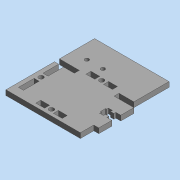
# Autodesk Inventor part: X-Anchor_Side
Saved by Autodesk Inventor 2016 SP1 (Build 200210100, 210)
## iProperties
Created: 2015-12-01
Part Number: X-Anchor_Side
Material: Generic
Document SubType Name: Modeling
Designer: Mohamed A.
Density: 1 g/cm^3
Appearance: Default
Author: Mohamed A.
Autodesk Inventor part; units mm, degrees
ref_plane "YZ Plane" through (0, 0, 0) normal (1, 0, 0) x (0, 1, 0)
ref_plane "XZ Plane" through (0, 0, 0) normal (0, 1, 0) x (-1, 0, 0)
ref_plane "XY Plane" through (0, 0, 0) normal (0, 0, 1) x (1, 0, 0)
sketch "Sketch1" plane through (0, 0, 0) normal (0, 0, 1) x (1, 0, 0)
  line L0 (0, 0) -> (47.5, 0)
  line L1 (47.5, 0) -> (47.5, 37)
  line L2 (47.5, 37) -> (0, 37)
  line L3 (0, 37) -> (0, 0)
  dimension "d60" = 47.5
  dimension "d61" = 37
  constraints: 8 end point, 2 parallel, 1 horizontal, 1 perpendicular
  measures "d60" distance between parallel lines of L1 L3
  measures "d61" distance between parallel lines of L0 L2
extrude "Extrusion1" add sketch "Sketch1" against normal blind 3
sketch "Sketch6" plane through (0, 0, 0) normal (0, 0, 1) x (1, 0, 0)
  line L0 (47.5, 0) -> (47.5, 37) projected
  line L1 (47.5, 37) -> (0, 37) projected
  line L2 (0, 37) -> (47.5, 37) projected
  line L3 (47.5, 37) -> (44.5, 37)
  line L4 (44.5, 37) -> (44.5, 29)
  line L5 (44.5, 29) -> (47.5, 29)
  line L6 (47.5, 29) -> (47.5, 37)
  line L7 (44.5, 0) -> (44.5, 8)
  line L8 (44.5, 8) -> (47.5, 8)
  line L9 (47.5, 8) -> (47.5, 0)
  line L10 (47.5, 0) -> (44.5, 0)
  line L11 (-10.772, 18.5) -> (61.9279, 18.5) construction
  line L12 (23.75, 42.476) -> (23.75, -8.8223) construction
  line L13 (47.5, 20) -> (39.5, 20)
  line L14 (39.5, 20) -> (39.5, 17)
  line L15 (39.5, 17) -> (47.5, 17)
  line L16 (47.5, 17) -> (47.5, 20)
  line L17 (47.5, 37) -> (47.5, 0) projected
  line L18 (44.5, 21.15) -> (47.5, 21.15)
  line L19 (47.5, 21.15) -> (47.5, 15.85)
  line L20 (47.5, 15.85) -> (44.5, 15.85)
  line L21 (44.5, 15.85) -> (44.5, 21.15)
  line L22 (40.1, 21.15) -> (42.5, 21.15)
  line L23 (42.5, 21.15) -> (42.5, 15.85)
  line L24 (42.5, 15.85) -> (40.1, 15.85)
  line L25 (40.1, 15.85) -> (40.1, 21.15)
  line L26 (15.8333, 35) -> (21.1, 35)
  line L27 (31.6667, 35) -> (31.6667, 32)
  line L28 (31.6667, 32) -> (26.4, 32)
  line L29 (15.8333, 32) -> (15.8333, 35)
  line L30 (26.4, 35) -> (26.4, 32)
  line L31 (21.1, 32) -> (21.1, 35)
  line L32 (26.4, 35) -> (31.6667, 35)
  line L33 (21.1, 32) -> (15.8333, 32)
  circle A0 centre (23.75, 33.5) radius 1.4
  line L34 (0, 0) -> (47.5, 0) projected
  line L35 (0, 0) -> (0, 37) projected
  line L36 (0, 32) -> (11.875, 32)
  line L37 (11.875, 32) -> (11.875, 29)
  line L38 (11.875, 29) -> (0, 29)
  line L39 (0, 29) -> (0, 32)
  line L40 (44.5, 32) -> (35.625, 32)
  line L41 (35.625, 32) -> (35.625, 29)
  line L42 (35.625, 29) -> (44.5, 29)
  line L43 (44.5, 29) -> (44.5, 32)
  line L44 (15.8333, 2) -> (21.1, 2)
  line L45 (31.6667, 2) -> (31.6667, 5)
  line L46 (31.6667, 5) -> (26.4, 5)
  line L47 (15.8333, 5) -> (15.8333, 2)
  line L48 (26.4, 2) -> (26.4, 5)
  line L49 (21.1, 5) -> (21.1, 2)
  line L50 (26.4, 2) -> (31.6667, 2)
  line L51 (21.1, 5) -> (15.8333, 5)
  circle A1 centre (23.75, 3.5) radius 1.4
  line L52 (5.5, 19.65) -> (2.5, 19.65)
  line L53 (2.5, 19.65) -> (2.5, 29)
  line L54 (2.5, 29) -> (5.5, 29)
  line L55 (5.5, 29) -> (5.5, 19.65)
  line L56 (2.5, 14.35) -> (5.5, 14.35)
  line L57 (5.5, 14.35) -> (5.5, 5)
  line L58 (5.5, 5) -> (2.5, 5)
  line L59 (2.5, 5) -> (2.5, 14.35)
  circle A2 centre (4, 17) radius 1.4
  dimension "d65" = 3
  dimension "d75" = 8
  dimension "d76" = 3
  dimension "d78" = 5.3
  dimension "d80" = 5
  dimension "d81" = 2.4
  dimension "d83" = 3
  dimension "d84" = 15.8333
  dimension "d85" = 2
  dimension "d86" = 5.3
  dimension "d87" = 2.8
  dimension "d88" = 3
  dimension "d89" = 23.75
  dimension "d90" = 47.5
  dimension "d91" = 2.8
  dimension "d92" = 5.3
  dimension "d93" = 2.65
  dimension "d94" = 1.5
  constraints: 108 end point, 20 parallel, 15 horizontal, 9 symmetric about line, 8 collinear, 8 point on line, 7 perpendicular, 6 vertical, 3 centre point, 16 other
  measures "d65" distance of L5.end L4.end
  measures "d75" distance of L15.end L14.end
  measures "d76" distance of L14.end L13.end
  measures "d78" distance between parallel lines of L20 L18
  measures "d80" distance between parallel lines of L0 L23
  measures "d81" distance between parallel lines of L25 L23
  measures "d83" distance of L27.start L27.end
  measures "d84" distance between parallel lines of L27 L29
  measures "d85" distance between parallel lines of L26 L1
  measures "d86" distance of L28.end L31.start
  measures "d87" diameter of A0
  measures "d88" distance of L36.end L37.end
  measures "d89" distance between parallel lines of L41 L37
  measures "d90" distance between parallel lines of L0 L35
  measures "d91" diameter of A2
  measures "d92" distance between parallel lines of L52 L56
  measures "d93" distance from line of A2.centre L56
  measures "d94" distance from line of L59 A2.centre
extrude "Extrusion6" cut sketch "Sketch6" against normal blind 3 contours L10 L7 L8 L0 | L20 L21 L15 L0 | L15 L21 L13 L0 | L35 L36 L37 L38 | L13 L21 L18 L0 | L15 L23 L13 L21 | L38 L55 L52 L53 | L23 L24 L25 L15 | L15 L25 L13 L23 | L5 L4 L1 L0 | L13 L25 L22 L23 | L15 L14 L13 L25 | L42 L41 L40 L4 | L26 L31 L33 L29 | L27 L28 L30 L32 | A0 | L47 L51 L49 L44 | L50 L48 L46 L45 | A1 | L56 L57 L58 L59 | A2
sketch "Sketch9" plane through (0, 37, 0) normal (0, 1, 0) x (1, 0, 0)
  line L0 (44.5, 0) -> (44.5, 3) projected
  line L1 (0, 3) -> (44.5, 3) projected
  line L2 (0, 0) -> (0, 3) projected
  line L3 (44.5, 0) -> (0, 0) projected
  point P0 (0, 0)
extrude "Extrusion8" add sketch "Sketch9" along normal blind 16
sketch "Sketch10" plane through (0, 0, 0) normal (0, 0, 1) x (1, 0, 0)
  circle A0 centre (8.6339, 43.7833) radius 1.1938
  circle A1 centre (18.1589, 43.7833) radius 1.1938
  line L0 (0, 53) -> (44.5, 53) projected
  point P0 (0, 0)
  dimension "d99" = 2.3876
  dimension "d100" = 2.3876
  dimension "d101" = 9.2167
  dimension "d102" = 9.2167
  constraints: 2 centre point
  measures "d99" diameter of A1
  measures "d100" diameter of A0
  measures "d101" distance from line of L0 A0.centre
  measures "d102" distance from line of A1.centre L0
extrude "Extrusion9" cut sketch "Sketch10" against normal up to next
equation "\"d89\" = 0.5 * d90"
equation "\"d93\" = 0.5 * d92"
equation "\"d102\" = d101"
equation "\"d15\" = 0.333333 * d14"
equation "\"d14\" = 30"
body "Solid1"
